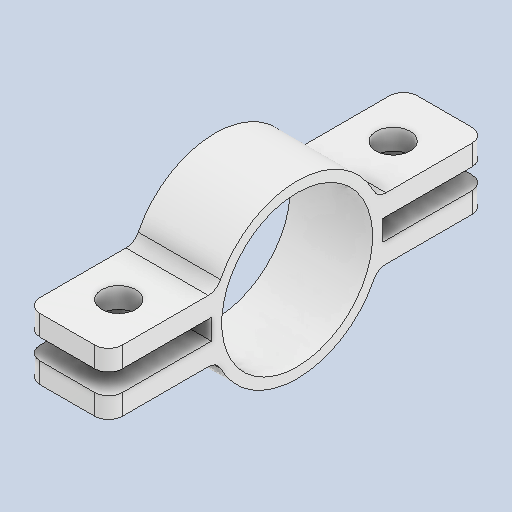
# Autodesk Inventor part: Abraçadeira_CPY1_CPY_CPY1
Saved by Autodesk Inventor 2024 (Build 280153000, 153)
## iProperties
Created: 2024-05-05
Part Number: Abraçadeira_CPY1_CPY_CPY1
Material: ABS plástico
Document SubType Name: Modeling
Designer: mathe
Density: 1.06 g/cm^3
Appearance: Suave - Branco
Author: mathe
Autodesk Inventor part; units mm, degrees
ref_plane "YZ Plane" through (0, 0, 0) normal (1, 0, 0) x (0, 1, 0)
ref_plane "XZ Plane" through (0, 0, 0) normal (0, 1, 0) x (-1, 0, 0)
ref_plane "XY Plane" through (0, 0, 0) normal (0, 0, 1) x (1, 0, 0)
sketch "Esboço1" plane through (0, 0, 0) normal (1, 0, 0) x (0, 1, 0)
  circle A0 centre (0, 0) radius 11
  line L0 (1.5, -27.5) -> (1.5, -12.4097)
  line L1 (1.5, 12.4097) -> (1.5, 27.5)
  line L2 (4.5, -27.5) -> (4.5, -11.6619)
  line L3 (4.5, 11.6619) -> (4.5, 27.5)
  line L4 (-4.5, 27.5) -> (-4.5, 11.6619)
  line L5 (-4.5, -11.6619) -> (-4.5, -27.5)
  line L6 (-1.5, 27.5) -> (-1.5, 12.4097)
  line L7 (-1.5, -12.4097) -> (-1.5, -27.5)
  line L8 (-4.5, -27.5) -> (-1.5, -27.5)
  line L9 (1.5, -27.5) -> (4.5, -27.5)
  line L10 (4.5, 27.5) -> (1.5, 27.5)
  line L11 (-1.5, 27.5) -> (-4.5, 27.5)
  line L12 (0, -12.5) -> (1.5, -12.5)
  line L13 (0, -12.5) -> (-1.5, -12.5)
  line L14 (0, 12.5) -> (1.5, 12.5)
  line L15 (0, 12.5) -> (-1.5, 12.5)
  arc A1 (-1.5, 12.4097) -> (-1.5, -12.4097) centre (0, 0) ccw
  arc A2 (1.5, -12.4097) -> (1.5, 12.4097) centre (0, 0) ccw
  dimension "d0" = 22
  constraints: 32 end point, 12 parallel, 8 point on circle, 6 perpendicular, 6 point on line, 3 centre point, 2 coincident, 2 horizontal, 1 tangent
  measures "d0" diameter of A0
extrude "Extrusão1" add sketch "Esboço1" along normal mid plane 12
sketch "Esboço2" plane through (-6, 4.5, 27.5) normal (0, 1, 0) x (1, 0, 0)
  point P0 (6, 27.5)
sketch "Esboço3" plane through (-6, -1.5, 27.5) normal (0, 1, 0) x (1, 0, 0)
  circle A0 centre (6, 7.5) radius 2.5
  line L0 (0, 0) -> (12, 0) projected
  line L1 (12, 15) -> (12, 0) projected
  line L2 (0, 0) -> (0, 15.8381) projected
  point P0 (6, 27.5)
  dimension "d17" = 5
  dimension "d18" = 7.5
  dimension "d19" = 6
  constraints: 1 centre point
  measures "d17" diameter of A0
  measures "d18" distance from line of L0 A0.centre
  measures "d19" distance from line of L1 A0.centre
hole "Furo1" at (0, -1.5, 20) direction (0, -1, 0) diameter 5 end through all both
sketch "Esboço4" plane through (-6, -1.5, -12.5) normal (0, 1, 0) x (1, 0, 0)
  circle A0 centre (6, 7.5) radius 2.5
  line L0 (12, 15) -> (0, 15) projected
  line L1 (12, 15) -> (12, -0.8381) projected
  point P0 (6, -12.5)
  dimension "d28" = 5
  dimension "d29" = 7.5
  dimension "d30" = 6
  constraints: 1 centre point
  measures "d28" diameter of A0
  measures "d29" distance from line of L0 A0.centre
  measures "d30" distance from line of L1 A0.centre
hole "Furo2" at (0, -1.5, -20) direction (0, -1, 0) diameter 5 end through all both
fillet "Arredondamento1" radius 2 12 edges at (0, 4.5, 11.6619) (0, 4.5, -11.6619) (0, -4.5, -11.6619) (0, -4.5, 11.6619) (6, 3, 27.5) (-6, 3, 27.5) (-6, -3, 27.5) (6, -3, 27.5) (6, 3, -27.5) (6, -3, -27.5) (-6, -3, -27.5) (-6, 3, -27.5)
